Autodesk Fusion 360 part; units mm, degrees
(part 6 of 6)
sketch "Sketch8" plane through (0, -4, 0) normal (0, -1, 0) x (1, 0, 0)
  line L0 (88.7705, -19.8875) -> (88.7705, -2.0326)
  line L1 (88.7705, -2.0326) -> (97.8711, -2.0326)
  line L2 (97.8711, -2.0326) -> (97.8711, -1.7823)
  line L3 (97.8711, -1.7823) -> (111.87, -1.7823)
  line L4 (111.87, -1.7823) -> (111.87, -2.0326)
  line L5 (111.87, -2.0326) -> (120.971, -2.0326)
  line L6 (120.971, -2.0326) -> (120.971, -19.8875)
  line L7 (120.971, -19.8875) -> (88.7705, -19.8875)
  line L8 (26.1455, -15.7827) -> (26.1455, -17.7817)
  line L9 (26.1455, -17.7817) -> (12.146, -17.7817)
  line L10 (12.146, -17.7817) -> (12.146, -15.7827)
  line L11 (12.146, -15.7827) -> (11.3454, -15.7827)
  line L12 (11.3454, -15.7827) -> (11.3454, -12.6821)
  line L13 (11.3454, -12.6821) -> (12.146, -12.6821)
  line L14 (12.146, -12.6821) -> (12.146, -6.8819)
  line L15 (12.146, -6.8819) -> (11.3454, -6.8819)
  line L16 (11.3454, -6.8819) -> (11.3454, -3.7827)
  line L17 (11.3454, -3.7827) -> (12.146, -3.7827)
  line L18 (12.146, -3.7827) -> (12.146, -1.7823)
  line L19 (12.146, -1.7823) -> (26.1455, -1.7823)
  line L20 (26.1455, -1.7823) -> (26.1455, -3.7827)
  line L21 (26.1455, -3.7827) -> (26.9462, -3.7827)
  line L22 (26.9462, -3.7827) -> (26.9462, -6.8819)
  line L23 (26.9462, -6.8819) -> (26.1455, -6.8819)
  line L24 (26.1455, -6.8819) -> (26.1455, -12.6821)
  line L25 (26.1455, -12.6821) -> (26.9462, -12.6821)
  line L26 (26.9462, -12.6821) -> (26.9462, -15.7827)
  line L27 (26.9462, -15.7827) -> (26.1455, -15.7827)
  line L28 (73.7704, -34.8327) -> (73.7704, -36.8316)
  line L29 (73.7704, -36.8316) -> (59.7711, -36.8316)
  line L30 (59.7711, -36.8316) -> (59.7711, -34.8327)
  line L31 (59.7711, -34.8327) -> (58.9703, -34.8327)
  line L32 (58.9703, -34.8327) -> (58.9703, -31.7321)
  line L33 (58.9703, -31.7321) -> (59.7711, -31.7321)
  line L34 (59.7711, -31.7321) -> (59.7711, -25.9319)
  line L35 (59.7711, -25.9319) -> (58.9703, -25.9319)
  line L36 (58.9703, -25.9319) -> (58.9703, -22.8327)
  line L37 (58.9703, -22.8327) -> (59.7711, -22.8327)
  line L38 (59.7711, -22.8327) -> (59.7711, -20.8323)
  line L39 (59.7711, -20.8323) -> (73.7704, -20.8323)
  line L40 (73.7704, -20.8323) -> (73.7704, -22.8327)
  line L41 (73.7704, -22.8327) -> (74.5712, -22.8327)
  line L42 (74.5712, -22.8327) -> (74.5712, -25.9319)
  line L43 (74.5712, -25.9319) -> (73.7704, -25.9319)
  line L44 (73.7704, -25.9319) -> (73.7704, -31.7321)
  line L45 (73.7704, -31.7321) -> (74.5712, -31.7321)
  line L46 (74.5712, -31.7321) -> (74.5712, -34.8327)
  line L47 (74.5712, -34.8327) -> (73.7704, -34.8327)
  line L48 (174.071, -41.8828) -> (174.071, -39.8824)
  line L49 (174.071, -39.8824) -> (188.07, -39.8824)
  line L50 (188.07, -39.8824) -> (188.07, -41.8828)
  line L51 (188.07, -41.8828) -> (188.871, -41.8828)
  line L52 (188.871, -41.8828) -> (188.871, -44.982)
  line L53 (188.871, -44.982) -> (188.07, -44.982)
  line L54 (188.07, -44.982) -> (188.07, -50.782)
  line L55 (188.07, -50.782) -> (188.871, -50.782)
  line L56 (188.871, -50.782) -> (188.871, -53.8826)
  line L57 (188.871, -53.8826) -> (188.07, -53.8826)
  line L58 (188.07, -53.8826) -> (188.07, -55.8816)
  line L59 (188.07, -55.8816) -> (174.071, -55.8816)
  line L60 (174.071, -55.8816) -> (174.071, -53.8826)
  line L61 (174.071, -53.8826) -> (173.27, -53.8826)
  line L62 (173.27, -53.8826) -> (173.27, -50.782)
  line L63 (173.27, -50.782) -> (174.071, -50.782)
  line L64 (174.071, -50.782) -> (174.071, -44.982)
  line L65 (174.071, -44.982) -> (173.27, -44.982)
  line L66 (173.27, -44.982) -> (173.27, -41.8828)
  line L67 (173.27, -41.8828) -> (174.071, -41.8828)
  line L68 (16.6205, -53.8826) -> (16.6205, -55.8816)
  line L69 (16.6205, -55.8816) -> (2.621, -55.8816)
  line L70 (2.621, -55.8816) -> (2.621, -53.8826)
  line L71 (2.621, -53.8826) -> (1.8204, -53.8826)
  line L72 (1.8204, -53.8826) -> (1.8204, -50.782)
  line L73 (1.8204, -50.782) -> (2.621, -50.782)
  line L74 (2.621, -50.782) -> (2.621, -44.982)
  line L75 (2.621, -44.982) -> (1.8204, -44.982)
  line L76 (1.8204, -44.982) -> (1.8204, -41.8828)
  line L77 (1.8204, -41.8828) -> (2.621, -41.8828)
  line L78 (2.621, -41.8828) -> (2.621, -39.8824)
  line L79 (2.621, -39.8824) -> (16.6205, -39.8824)
  line L80 (16.6205, -39.8824) -> (16.6205, -41.8828)
  line L81 (16.6205, -41.8828) -> (17.4212, -41.8828)
  line L82 (17.4212, -41.8828) -> (17.4212, -44.982)
  line L83 (17.4212, -44.982) -> (16.6205, -44.982)
  line L84 (16.6205, -44.982) -> (16.6205, -50.782)
  line L85 (16.6205, -50.782) -> (17.4212, -50.782)
  line L86 (17.4212, -50.782) -> (17.4212, -53.8826)
  line L87 (17.4212, -53.8826) -> (16.6205, -53.8826)
  line L88 (59.7711, -41.8828) -> (59.7711, -39.8824)
  line L89 (59.7711, -39.8824) -> (73.7704, -39.8824)
  line L90 (73.7704, -39.8824) -> (73.7704, -41.8828)
  line L91 (73.7704, -41.8828) -> (74.5712, -41.8828)
  line L92 (74.5712, -41.8828) -> (74.5712, -44.982)
  line L93 (74.5712, -44.982) -> (73.7704, -44.982)
  line L94 (73.7704, -44.982) -> (73.7704, -50.782)
  line L95 (73.7704, -50.782) -> (74.5712, -50.782)
  line L96 (74.5712, -50.782) -> (74.5712, -53.8826)
  line L97 (74.5712, -53.8826) -> (73.7704, -53.8826)
  line L98 (73.7704, -53.8826) -> (73.7704, -55.8816)
  line L99 (73.7704, -55.8816) -> (59.7711, -55.8816)
  line L100 (59.7711, -55.8816) -> (59.7711, -53.8826)
  line L101 (59.7711, -53.8826) -> (58.9703, -53.8826)
  line L102 (58.9703, -53.8826) -> (58.9703, -50.782)
  line L103 (58.9703, -50.782) -> (59.7711, -50.782)
  line L104 (59.7711, -50.782) -> (59.7711, -44.982)
  line L105 (59.7711, -44.982) -> (58.9703, -44.982)
  line L106 (58.9703, -44.982) -> (58.9703, -41.8828)
  line L107 (58.9703, -41.8828) -> (59.7711, -41.8828)
  line L108 (135.971, -41.8828) -> (135.971, -39.8824)
  line L109 (135.971, -39.8824) -> (149.97, -39.8824)
  line L110 (149.97, -39.8824) -> (149.97, -41.8828)
  line L111 (149.97, -41.8828) -> (150.771, -41.8828)
  line L112 (150.771, -41.8828) -> (150.771, -44.982)
  line L113 (150.771, -44.982) -> (149.97, -44.982)
  line L114 (149.97, -44.982) -> (149.97, -50.782)
  line L115 (149.97, -50.782) -> (150.771, -50.782)
  line L116 (150.771, -50.782) -> (150.771, -53.8826)
  line L117 (150.771, -53.8826) -> (149.97, -53.8826)
  line L118 (149.97, -53.8826) -> (149.97, -55.8816)
  line L119 (149.97, -55.8816) -> (135.971, -55.8816)
  line L120 (135.971, -55.8816) -> (135.971, -53.8826)
  line L121 (135.971, -53.8826) -> (135.17, -53.8826)
  line L122 (135.17, -53.8826) -> (135.17, -50.782)
  line L123 (135.17, -50.782) -> (135.971, -50.782)
  line L124 (135.971, -50.782) -> (135.971, -44.982)
  line L125 (135.971, -44.982) -> (135.17, -44.982)
  line L126 (135.17, -44.982) -> (135.17, -41.8828)
  line L127 (135.17, -41.8828) -> (135.971, -41.8828)
  line L128 (92.8204, -53.8826) -> (92.8204, -55.8816)
  line L129 (92.8204, -55.8816) -> (78.8211, -55.8816)
  line L130 (78.8211, -55.8816) -> (78.8211, -53.8826)
  line L131 (78.8211, -53.8826) -> (78.0203, -53.8826)
  line L132 (78.0203, -53.8826) -> (78.0203, -50.782)
  line L133 (78.0203, -50.782) -> (78.8211, -50.782)
  line L134 (78.8211, -50.782) -> (78.8211, -44.982)
  line L135 (78.8211, -44.982) -> (78.0203, -44.982)
  line L136 (78.0203, -44.982) -> (78.0203, -41.8828)
  line L137 (78.0203, -41.8828) -> (78.8211, -41.8828)
  line L138 (78.8211, -41.8828) -> (78.8211, -39.8824)
  line L139 (78.8211, -39.8824) -> (92.8204, -39.8824)
  line L140 (92.8204, -39.8824) -> (92.8204, -41.8828)
  line L141 (92.8204, -41.8828) -> (93.6198, -41.8828)
  line L142 (93.6198, -41.8828) -> (93.6198, -44.982)
  line L143 (93.6198, -44.982) -> (92.8204, -44.982)
  line L144 (92.8204, -44.982) -> (92.8204, -50.782)
  line L145 (92.8204, -50.782) -> (93.6198, -50.782)
  line L146 (93.6198, -50.782) -> (93.6198, -53.8826)
  line L147 (93.6198, -53.8826) -> (92.8204, -53.8826)
  line L148 (126.446, -3.7827) -> (126.446, -1.7823)
  line L149 (126.446, -1.7823) -> (140.445, -1.7823)
  line L150 (140.445, -1.7823) -> (140.445, -3.7827)
  line L151 (140.445, -3.7827) -> (141.246, -3.7827)
  line L152 (141.246, -3.7827) -> (141.246, -6.8819)
  line L153 (141.246, -6.8819) -> (140.445, -6.8819)
  line L154 (140.445, -6.8819) -> (140.445, -12.6821)
  line L155 (140.445, -12.6821) -> (141.246, -12.6821)
  line L156 (141.246, -12.6821) -> (141.246, -15.7827)
  line L157 (141.246, -15.7827) -> (140.445, -15.7827)
  line L158 (140.445, -15.7827) -> (140.445, -17.7817)
  line L159 (140.445, -17.7817) -> (126.446, -17.7817)
  line L160 (126.446, -17.7817) -> (126.446, -15.7827)
  line L161 (126.446, -15.7827) -> (125.645, -15.7827)
  line L162 (125.645, -15.7827) -> (125.645, -12.6821)
  line L163 (125.645, -12.6821) -> (126.446, -12.6821)
  line L164 (126.446, -12.6821) -> (126.446, -6.8819)
  line L165 (126.446, -6.8819) -> (125.645, -6.8819)
  line L166 (125.645, -6.8819) -> (125.645, -3.7827)
  line L167 (125.645, -3.7827) -> (126.446, -3.7827)
  line L168 (64.2454, -1.7823) -> (64.2454, -3.7827)
  line L169 (64.2454, -3.7827) -> (65.0462, -3.7827)
  line L170 (65.0462, -3.7827) -> (65.0462, -6.8819)
  line L171 (65.0462, -6.8819) -> (64.2454, -6.8819)
  line L172 (64.2454, -6.8819) -> (64.2454, -12.6821)
  line L173 (64.2454, -12.6821) -> (65.0462, -12.6821)
  line L174 (65.0462, -12.6821) -> (65.0462, -15.7827)
  line L175 (65.0462, -15.7827) -> (64.2454, -15.7827)
  line L176 (64.2454, -15.7827) -> (64.2454, -17.7817)
  line L177 (64.2454, -17.7817) -> (50.2461, -17.7817)
  line L178 (50.2461, -17.7817) -> (50.2461, -15.7827)
  line L179 (50.2461, -15.7827) -> (49.4453, -15.7827)
  line L180 (49.4453, -15.7827) -> (49.4453, -12.6821)
  line L181 (49.4453, -12.6821) -> (50.2461, -12.6821)
  line L182 (50.2461, -12.6821) -> (50.2461, -6.8819)
  line L183 (50.2461, -6.8819) -> (49.4453, -6.8819)
  line L184 (49.4453, -6.8819) -> (49.4453, -3.7827)
  line L185 (49.4453, -3.7827) -> (50.2461, -3.7827)
  line L186 (50.2461, -3.7827) -> (50.2461, -1.7823)
  line L187 (50.2461, -1.7823) -> (64.2454, -1.7823)
  line L188 (164.546, -17.7817) -> (164.546, -15.7827)
  line L189 (164.546, -15.7827) -> (163.745, -15.7827)
  line L190 (163.745, -15.7827) -> (163.745, -12.6821)
  line L191 (163.745, -12.6821) -> (164.546, -12.6821)
  line L192 (164.546, -12.6821) -> (164.546, -6.8819)
  line L193 (164.546, -6.8819) -> (163.745, -6.8819)
  line L194 (163.745, -6.8819) -> (163.745, -3.7827)
  line L195 (163.745, -3.7827) -> (164.546, -3.7827)
  line L196 (164.546, -3.7827) -> (164.546, -1.7823)
  line L197 (164.546, -1.7823) -> (178.545, -1.7823)
  line L198 (178.545, -1.7823) -> (178.545, -3.7827)
  line L199 (178.545, -3.7827) -> (179.346, -3.7827)
  line L200 (179.346, -3.7827) -> (179.346, -6.8819)
  line L201 (179.346, -6.8819) -> (178.545, -6.8819)
  line L202 (178.545, -6.8819) -> (178.545, -12.6821)
  line L203 (178.545, -12.6821) -> (179.346, -12.6821)
  line L204 (179.346, -12.6821) -> (179.346, -15.7827)
  line L205 (179.346, -15.7827) -> (178.545, -15.7827)
  line L206 (178.545, -15.7827) -> (178.545, -17.7817)
  line L207 (178.545, -17.7817) -> (164.546, -17.7817)
  line L208 (69.2961, -17.7817) -> (69.2961, -15.7827)
  line L209 (69.2961, -15.7827) -> (68.4953, -15.7827)
  line L210 (68.4953, -15.7827) -> (68.4953, -12.6821)
  line L211 (68.4953, -12.6821) -> (69.2961, -12.6821)
  line L212 (69.2961, -12.6821) -> (69.2961, -6.8819)
  line L213 (69.2961, -6.8819) -> (68.4953, -6.8819)
  line L214 (68.4953, -6.8819) -> (68.4953, -3.7827)
  line L215 (68.4953, -3.7827) -> (69.2961, -3.7827)
  line L216 (69.2961, -3.7827) -> (69.2961, -1.7823)
  line L217 (69.2961, -1.7823) -> (83.2954, -1.7823)
  line L218 (83.2954, -1.7823) -> (83.2954, -3.7827)
  line L219 (83.2954, -3.7827) -> (84.0962, -3.7827)
  line L220 (84.0962, -3.7827) -> (84.0962, -6.8819)
  line L221 (84.0962, -6.8819) -> (83.2954, -6.8819)
  line L222 (83.2954, -6.8819) -> (83.2954, -12.6821)
  line L223 (83.2954, -12.6821) -> (84.0962, -12.6821)
  line L224 (84.0962, -12.6821) -> (84.0962, -15.7827)
  line L225 (84.0962, -15.7827) -> (83.2954, -15.7827)
  line L226 (83.2954, -15.7827) -> (83.2954, -17.7817)
  line L227 (83.2954, -17.7817) -> (69.2961, -17.7817)
  line L228 (188.07, -20.8323) -> (188.07, -22.8327)
  line L229 (188.07, -22.8327) -> (188.871, -22.8327)
  line L230 (188.871, -22.8327) -> (188.871, -25.9319)
  line L231 (188.871, -25.9319) -> (188.07, -25.9319)
  line L232 (188.07, -25.9319) -> (188.07, -31.7321)
  line L233 (188.07, -31.7321) -> (188.871, -31.7321)
  line L234 (188.871, -31.7321) -> (188.871, -34.8327)
  line L235 (188.871, -34.8327) -> (188.07, -34.8327)
  line L236 (188.07, -34.8327) -> (188.07, -36.8316)
  line L237 (188.07, -36.8316) -> (174.071, -36.8316)
  line L238 (174.071, -36.8316) -> (174.071, -34.8327)
  line L239 (174.071, -34.8327) -> (173.27, -34.8327)
  line L240 (173.27, -34.8327) -> (173.27, -31.7321)
  line L241 (173.27, -31.7321) -> (174.071, -31.7321)
  line L242 (174.071, -31.7321) -> (174.071, -25.9319)
  line L243 (174.071, -25.9319) -> (173.27, -25.9319)
  line L244 (173.27, -25.9319) -> (173.27, -22.8327)
  line L245 (173.27, -22.8327) -> (174.071, -22.8327)
  line L246 (174.071, -22.8327) -> (174.071, -20.8323)
  line L247 (174.071, -20.8323) -> (188.07, -20.8323)
  line L248 (130.92, -39.8824) -> (130.92, -41.8828)
  line L249 (130.92, -41.8828) -> (131.721, -41.8828)
  line L250 (131.721, -41.8828) -> (131.721, -44.982)
  line L251 (131.721, -44.982) -> (130.92, -44.982)
  line L252 (130.92, -44.982) -> (130.92, -50.782)
  line L253 (130.92, -50.782) -> (131.721, -50.782)
  line L254 (131.721, -50.782) -> (131.721, -53.8826)
  line L255 (131.721, -53.8826) -> (130.92, -53.8826)
  line L256 (130.92, -53.8826) -> (130.92, -55.8816)
  line L257 (130.92, -55.8816) -> (116.92, -55.8816)
  line L258 (116.92, -55.8816) -> (116.92, -53.8826)
  line L259 (116.92, -53.8826) -> (116.119, -53.8826)
  line L260 (116.119, -53.8826) -> (116.119, -50.782)
  line L261 (116.119, -50.782) -> (116.92, -50.782)
  line L262 (116.92, -50.782) -> (116.92, -44.982)
  line L263 (116.92, -44.982) -> (116.119, -44.982)
  line L264 (116.119, -44.982) -> (116.119, -41.8828)
  line L265 (116.119, -41.8828) -> (116.92, -41.8828)
  line L266 (116.92, -41.8828) -> (116.92, -39.8824)
  line L267 (116.92, -39.8824) -> (130.92, -39.8824)
  line L268 (92.8204, -20.8323) -> (92.8204, -22.8327)
  line L269 (92.8204, -22.8327) -> (93.6198, -22.8327)
  line L270 (93.6198, -22.8327) -> (93.6198, -25.9319)
  line L271 (93.6198, -25.9319) -> (92.8204, -25.9319)
  line L272 (92.8204, -25.9319) -> (92.8204, -31.7321)
  line L273 (92.8204, -31.7321) -> (93.6198, -31.7321)
  line L274 (93.6198, -31.7321) -> (93.6198, -34.8327)
  line L275 (93.6198, -34.8327) -> (92.8204, -34.8327)
  line L276 (92.8204, -34.8327) -> (92.8204, -36.8316)
  line L277 (92.8204, -36.8316) -> (78.8211, -36.8316)
  line L278 (78.8211, -36.8316) -> (78.8211, -34.8327)
  line L279 (78.8211, -34.8327) -> (78.0203, -34.8327)
  line L280 (78.0203, -34.8327) -> (78.0203, -31.7321)
  line L281 (78.0203, -31.7321) -> (78.8211, -31.7321)
  line L282 (78.8211, -31.7321) -> (78.8211, -25.9319)
  line L283 (78.8211, -25.9319) -> (78.0203, -25.9319)
  line L284 (78.0203, -25.9319) -> (78.0203, -22.8327)
  line L285 (78.0203, -22.8327) -> (78.8211, -22.8327)
  line L286 (78.8211, -22.8327) -> (78.8211, -20.8323)
  line L287 (78.8211, -20.8323) -> (92.8204, -20.8323)
  line L288 (54.7204, -39.8824) -> (54.7204, -41.8828)
  line L289 (54.7204, -41.8828) -> (55.5212, -41.8828)
  line L290 (55.5212, -41.8828) -> (55.5212, -44.982)
  line L291 (55.5212, -44.982) -> (54.7204, -44.982)
  line L292 (54.7204, -44.982) -> (54.7204, -50.782)
  line L293 (54.7204, -50.782) -> (55.5212, -50.782)
  line L294 (55.5212, -50.782) -> (55.5212, -53.8826)
  line L295 (55.5212, -53.8826) -> (54.7204, -53.8826)
  line L296 (54.7204, -53.8826) -> (54.7204, -55.8816)
  line L297 (54.7204, -55.8816) -> (40.7211, -55.8816)
  line L298 (40.7211, -55.8816) -> (40.7211, -53.8826)
  line L299 (40.7211, -53.8826) -> (39.9203, -53.8826)
  line L300 (39.9203, -53.8826) -> (39.9203, -50.782)
  line L301 (39.9203, -50.782) -> (40.7211, -50.782)
  line L302 (40.7211, -50.782) -> (40.7211, -44.982)
  line L303 (40.7211, -44.982) -> (39.9203, -44.982)
  line L304 (39.9203, -44.982) -> (39.9203, -41.8828)
  line L305 (39.9203, -41.8828) -> (40.7211, -41.8828)
  line L306 (40.7211, -41.8828) -> (40.7211, -39.8824)
  line L307 (40.7211, -39.8824) -> (54.7204, -39.8824)
  line L308 (97.8697, -55.8816) -> (97.8697, -53.8826)
  line L309 (97.8697, -53.8826) -> (97.0703, -53.8826)
  line L310 (97.0703, -53.8826) -> (97.0703, -50.782)
  line L311 (97.0703, -50.782) -> (97.8697, -50.782)
  line L312 (97.8697, -50.782) -> (97.8697, -44.982)
  line L313 (97.8697, -44.982) -> (97.0703, -44.982)
  line L314 (97.0703, -44.982) -> (97.0703, -41.8828)
  line L315 (97.0703, -41.8828) -> (97.8697, -41.8828)
  line L316 (97.8697, -41.8828) -> (97.8697, -39.8824)
  line L317 (97.8697, -39.8824) -> (111.869, -39.8824)
  line L318 (111.869, -39.8824) -> (111.869, -41.8828)
  line L319 (111.869, -41.8828) -> (112.67, -41.8828)
  line L320 (112.67, -41.8828) -> (112.67, -44.982)
  line L321 (112.67, -44.982) -> (111.869, -44.982)
  line L322 (111.869, -44.982) -> (111.869, -50.782)
  line L323 (111.869, -50.782) -> (112.67, -50.782)
  line L324 (112.67, -50.782) -> (112.67, -53.8826)
  line L325 (112.67, -53.8826) -> (111.869, -53.8826)
  line L326 (111.869, -53.8826) -> (111.869, -55.8816)
  line L327 (111.869, -55.8816) -> (97.8697, -55.8816)
  line L328 (21.671, -55.8816) -> (21.671, -53.8826)
  line L329 (21.671, -53.8826) -> (20.8704, -53.8826)
  line L330 (20.8704, -53.8826) -> (20.8704, -50.782)
  line L331 (20.8704, -50.782) -> (21.671, -50.782)
  line L332 (21.671, -50.782) -> (21.671, -44.982)
  line L333 (21.671, -44.982) -> (20.8704, -44.982)
  line L334 (20.8704, -44.982) -> (20.8704, -41.8828)
  line L335 (20.8704, -41.8828) -> (21.671, -41.8828)
  line L336 (21.671, -41.8828) -> (21.671, -39.8824)
  line L337 (21.671, -39.8824) -> (35.6704, -39.8824)
  line L338 (35.6704, -39.8824) -> (35.6704, -41.8828)
  line L339 (35.6704, -41.8828) -> (36.4712, -41.8828)
  line L340 (36.4712, -41.8828) -> (36.4712, -44.982)
  line L341 (36.4712, -44.982) -> (35.6704, -44.982)
  line L342 (35.6704, -44.982) -> (35.6704, -50.782)
  line L343 (35.6704, -50.782) -> (36.4712, -50.782)
  line L344 (36.4712, -50.782) -> (36.4712, -53.8826)
  line L345 (36.4712, -53.8826) -> (35.6704, -53.8826)
  line L346 (35.6704, -53.8826) -> (35.6704, -55.8816)
  line L347 (35.6704, -55.8816) -> (21.671, -55.8816)
  line L348 (16.6205, -20.8323) -> (16.6205, -22.8327)
  line L349 (16.6205, -22.8327) -> (17.4212, -22.8327)
  line L350 (17.4212, -22.8327) -> (17.4212, -25.9319)
  line L351 (17.4212, -25.9319) -> (16.6205, -25.9319)
  line L352 (16.6205, -25.9319) -> (16.6205, -31.7321)
  line L353 (16.6205, -31.7321) -> (17.4212, -31.7321)
  line L354 (17.4212, -31.7321) -> (17.4212, -34.8327)
  line L355 (17.4212, -34.8327) -> (16.6205, -34.8327)
  line L356 (16.6205, -34.8327) -> (16.6205, -36.8316)
  line L357 (16.6205, -36.8316) -> (2.621, -36.8316)
  line L358 (2.621, -36.8316) -> (2.621, -34.8327)
  line L359 (2.621, -34.8327) -> (1.8204, -34.8327)
  line L360 (1.8204, -34.8327) -> (1.8204, -31.7321)
  line L361 (1.8204, -31.7321) -> (2.621, -31.7321)
  line L362 (2.621, -31.7321) -> (2.621, -25.9319)
  line L363 (2.621, -25.9319) -> (1.8204, -25.9319)
  line L364 (1.8204, -25.9319) -> (1.8204, -22.8327)
  line L365 (1.8204, -22.8327) -> (2.621, -22.8327)
  line L366 (2.621, -22.8327) -> (2.621, -20.8323)
  line L367 (2.621, -20.8323) -> (16.6205, -20.8323)
  line L368 (155.021, -55.8816) -> (155.021, -53.8826)
  line L369 (155.021, -53.8826) -> (154.22, -53.8826)
  line L370 (154.22, -53.8826) -> (154.22, -50.782)
  line L371 (154.22, -50.782) -> (155.021, -50.782)
  line L372 (155.021, -50.782) -> (155.021, -44.982)
  line L373 (155.021, -44.982) -> (154.22, -44.982)
  line L374 (154.22, -44.982) -> (154.22, -41.8828)
  line L375 (154.22, -41.8828) -> (155.021, -41.8828)
  line L376 (155.021, -41.8828) -> (155.021, -39.8824)
  line L377 (155.021, -39.8824) -> (169.02, -39.8824)
  line L378 (169.02, -39.8824) -> (169.02, -41.8828)
  line L379 (169.02, -41.8828) -> (169.821, -41.8828)
  line L380 (169.821, -41.8828) -> (169.821, -44.982)
  line L381 (169.821, -44.982) -> (169.02, -44.982)
  line L382 (169.02, -44.982) -> (169.02, -50.782)
  line L383 (169.02, -50.782) -> (169.821, -50.782)
  line L384 (169.821, -50.782) -> (169.821, -53.8826)
  line L385 (169.821, -53.8826) -> (169.02, -53.8826)
  line L386 (169.02, -53.8826) -> (169.02, -55.8816)
  line L387 (169.02, -55.8816) -> (155.021, -55.8816)
  line L388 (35.6704, -20.8323) -> (35.6704, -22.8327)
  line L389 (35.6704, -22.8327) -> (36.4712, -22.8327)
  line L390 (36.4712, -22.8327) -> (36.4712, -25.9319)
  line L391 (36.4712, -25.9319) -> (35.6704, -25.9319)
  line L392 (35.6704, -25.9319) -> (35.6704, -31.7321)
  line L393 (35.6704, -31.7321) -> (36.4712, -31.7321)
  line L394 (36.4712, -31.7321) -> (36.4712, -34.8327)
  line L395 (36.4712, -34.8327) -> (35.6704, -34.8327)
  line L396 (35.6704, -34.8327) -> (35.6704, -36.8316)
  line L397 (35.6704, -36.8316) -> (21.671, -36.8316)
  line L398 (21.671, -36.8316) -> (21.671, -34.8327)
  line L399 (21.671, -34.8327) -> (20.8704, -34.8327)
  line L400 (20.8704, -34.8327) -> (20.8704, -31.7321)
  line L401 (20.8704, -31.7321) -> (21.671, -31.7321)
  line L402 (21.671, -31.7321) -> (21.671, -25.9319)
  line L403 (21.671, -25.9319) -> (20.8704, -25.9319)
  line L404 (20.8704, -25.9319) -> (20.8704, -22.8327)
  line L405 (20.8704, -22.8327) -> (21.671, -22.8327)
  line L406 (21.671, -22.8327) -> (21.671, -20.8323)
  line L407 (21.671, -20.8323) -> (35.6704, -20.8323)
  line L408 (40.7211, -36.8316) -> (40.7211, -34.8327)
  line L409 (40.7211, -34.8327) -> (39.9203, -34.8327)
  line L410 (39.9203, -34.8327) -> (39.9203, -31.7321)
  line L411 (39.9203, -31.7321) -> (40.7211, -31.7321)
  line L412 (40.7211, -31.7321) -> (40.7211, -25.9319)
  line L413 (40.7211, -25.9319) -> (39.9203, -25.9319)
  line L414 (39.9203, -25.9319) -> (39.9203, -22.8327)
  line L415 (39.9203, -22.8327) -> (40.7211, -22.8327)
  line L416 (40.7211, -22.8327) -> (40.7211, -20.8323)
  line L417 (40.7211, -20.8323) -> (54.7204, -20.8323)
  line L418 (54.7204, -20.8323) -> (54.7204, -22.8327)
  line L419 (54.7204, -22.8327) -> (55.5212, -22.8327)
  line L420 (55.5212, -22.8327) -> (55.5212, -25.9319)
  line L421 (55.5212, -25.9319) -> (54.7204, -25.9319)
  line L422 (54.7204, -25.9319) -> (54.7204, -31.7321)
  line L423 (54.7204, -31.7321) -> (55.5212, -31.7321)
  line L424 (55.5212, -31.7321) -> (55.5212, -34.8327)
  line L425 (55.5212, -34.8327) -> (54.7204, -34.8327)
  line L426 (54.7204, -34.8327) -> (54.7204, -36.8316)
  line L427 (54.7204, -36.8316) -> (40.7211, -36.8316)
  line L428 (111.869, -20.8323) -> (111.869, -22.8327)
  line L429 (111.869, -22.8327) -> (112.67, -22.8327)
  line L430 (112.67, -22.8327) -> (112.67, -25.9319)
  line L431 (112.67, -25.9319) -> (111.869, -25.9319)
  line L432 (111.869, -25.9319) -> (111.869, -31.7321)
  line L433 (111.869, -31.7321) -> (112.67, -31.7321)
  line L434 (112.67, -31.7321) -> (112.67, -34.8327)
  line L435 (112.67, -34.8327) -> (111.869, -34.8327)
  line L436 (111.869, -34.8327) -> (111.869, -36.8316)
  line L437 (111.869, -36.8316) -> (97.8697, -36.8316)
  line L438 (97.8697, -36.8316) -> (97.8697, -34.8327)
  line L439 (97.8697, -34.8327) -> (97.0703, -34.8327)
  line L440 (97.0703, -34.8327) -> (97.0703, -31.7321)
  line L441 (97.0703, -31.7321) -> (97.8697, -31.7321)
  line L442 (97.8697, -31.7321) -> (97.8697, -25.9319)
  line L443 (97.8697, -25.9319) -> (97.0703, -25.9319)
  line L444 (97.0703, -25.9319) -> (97.0703, -22.8327)
  line L445 (97.0703, -22.8327) -> (97.8697, -22.8327)
  line L446 (97.8697, -22.8327) -> (97.8697, -20.8323)
  line L447 (97.8697, -20.8323) -> (111.869, -20.8323)
  line L448 (116.92, -36.8316) -> (116.92, -34.8327)
  line L449 (116.92, -34.8327) -> (116.119, -34.8327)
  line L450 (116.119, -34.8327) -> (116.119, -31.7321)
  line L451 (116.119, -31.7321) -> (116.92, -31.7321)
  line L452 (116.92, -31.7321) -> (116.92, -25.9319)
  line L453 (116.92, -25.9319) -> (116.119, -25.9319)
  line L454 (116.119, -25.9319) -> (116.119, -22.8327)
  line L455 (116.119, -22.8327) -> (116.92, -22.8327)
  line L456 (116.92, -22.8327) -> (116.92, -20.8323)
  line L457 (116.92, -20.8323) -> (130.92, -20.8323)
  line L458 (130.92, -20.8323) -> (130.92, -22.8327)
  line L459 (130.92, -22.8327) -> (131.721, -22.8327)
  line L460 (131.721, -22.8327) -> (131.721, -25.9319)
  line L461 (131.721, -25.9319) -> (130.92, -25.9319)
  line L462 (130.92, -25.9319) -> (130.92, -31.7321)
  line L463 (130.92, -31.7321) -> (131.721, -31.7321)
  line L464 (131.721, -31.7321) -> (131.721, -34.8327)
  line L465 (131.721, -34.8327) -> (130.92, -34.8327)
  line L466 (130.92, -34.8327) -> (130.92, -36.8316)
  line L467 (130.92, -36.8316) -> (116.92, -36.8316)
  line L468 (135.971, -36.8316) -> (135.971, -34.8327)
  line L469 (135.971, -34.8327) -> (135.17, -34.8327)
  line L470 (135.17, -34.8327) -> (135.17, -31.7321)
  line L471 (135.17, -31.7321) -> (135.971, -31.7321)
  line L472 (135.971, -31.7321) -> (135.971, -25.9319)
  line L473 (135.971, -25.9319) -> (135.17, -25.9319)
  line L474 (135.17, -25.9319) -> (135.17, -22.8327)
  line L475 (135.17, -22.8327) -> (135.971, -22.8327)
  line L476 (135.971, -22.8327) -> (135.971, -20.8323)
  line L477 (135.971, -20.8323) -> (149.97, -20.8323)
  line L478 (149.97, -20.8323) -> (149.97, -22.8327)
  line L479 (149.97, -22.8327) -> (150.771, -22.8327)
  line L480 (150.771, -22.8327) -> (150.771, -25.9319)
  line L481 (150.771, -25.9319) -> (149.97, -25.9319)
  line L482 (149.97, -25.9319) -> (149.97, -31.7321)
  line L483 (149.97, -31.7321) -> (150.771, -31.7321)
  line L484 (150.771, -31.7321) -> (150.771, -34.8327)
  line L485 (150.771, -34.8327) -> (149.97, -34.8327)
  line L486 (149.97, -34.8327) -> (149.97, -36.8316)
  line L487 (149.97, -36.8316) -> (135.971, -36.8316)
  line L488 (155.021, -36.8316) -> (155.021, -34.8327)
  line L489 (155.021, -34.8327) -> (154.22, -34.8327)
  line L490 (154.22, -34.8327) -> (154.22, -31.7321)
  line L491 (154.22, -31.7321) -> (155.021, -31.7321)
  line L492 (155.021, -31.7321) -> (155.021, -25.9319)
  line L493 (155.021, -25.9319) -> (154.22, -25.9319)
  line L494 (154.22, -25.9319) -> (154.22, -22.8327)
  line L495 (154.22, -22.8327) -> (155.021, -22.8327)
  line L496 (155.021, -22.8327) -> (155.021, -20.8323)
  line L497 (155.021, -20.8323) -> (169.02, -20.8323)
  line L498 (169.02, -20.8323) -> (169.02, -22.8327)
  line L499 (169.02, -22.8327) -> (169.821, -22.8327)
  line L500 (169.821, -22.8327) -> (169.821, -25.9319)
  line L501 (169.821, -25.9319) -> (169.02, -25.9319)
  line L502 (169.02, -25.9319) -> (169.02, -31.7321)
  line L503 (169.02, -31.7321) -> (169.821, -31.7321)
  line L504 (169.821, -31.7321) -> (169.821, -34.8327)
  line L505 (169.821, -34.8327) -> (169.02, -34.8327)
  line L506 (169.02, -34.8327) -> (169.02, -36.8316)
  line L507 (169.02, -36.8316) -> (155.021, -36.8316)
  line L508 (31.196, -3.7827) -> (31.196, -1.7823)
  line L509 (31.196, -1.7823) -> (45.1954, -1.7823)
  line L510 (45.1954, -1.7823) -> (45.1954, -3.7827)
  line L511 (45.1954, -3.7827) -> (45.9962, -3.7827)
  line L512 (45.9962, -3.7827) -> (45.9962, -6.8819)
  line L513 (45.9962, -6.8819) -> (45.1954, -6.8819)
  line L514 (45.1954, -6.8819) -> (45.1954, -12.6821)
  line L515 (45.1954, -12.6821) -> (45.9962, -12.6821)
  line L516 (45.9962, -12.6821) -> (45.9962, -15.7827)
  line L517 (45.9962, -15.7827) -> (45.1954, -15.7827)
  line L518 (45.1954, -15.7827) -> (45.1954, -17.7817)
  line L519 (45.1954, -17.7817) -> (31.196, -17.7817)
  line L520 (31.196, -17.7817) -> (31.196, -15.7827)
  line L521 (31.196, -15.7827) -> (30.3954, -15.7827)
  line L522 (30.3954, -15.7827) -> (30.3954, -12.6821)
  line L523 (30.3954, -12.6821) -> (31.196, -12.6821)
  line L524 (31.196, -12.6821) -> (31.196, -6.8819)
  line L525 (31.196, -6.8819) -> (30.3954, -6.8819)
  line L526 (30.3954, -6.8819) -> (30.3954, -3.7827)
  line L527 (30.3954, -3.7827) -> (31.196, -3.7827)
  line L528 (159.495, -1.7823) -> (159.495, -3.7827)
  line L529 (159.495, -3.7827) -> (160.296, -3.7827)
  line L530 (160.296, -3.7827) -> (160.296, -6.8819)
  line L531 (160.296, -6.8819) -> (159.495, -6.8819)
  line L532 (159.495, -6.8819) -> (159.495, -12.6821)
  line L533 (159.495, -12.6821) -> (160.296, -12.6821)
  line L534 (160.296, -12.6821) -> (160.296, -15.7827)
  line L535 (160.296, -15.7827) -> (159.495, -15.7827)
  line L536 (159.495, -15.7827) -> (159.495, -17.7817)
  line L537 (159.495, -17.7817) -> (145.496, -17.7817)
  line L538 (145.496, -17.7817) -> (145.496, -15.7827)
  line L539 (145.496, -15.7827) -> (144.695, -15.7827)
  line L540 (144.695, -15.7827) -> (144.695, -12.6821)
  line L541 (144.695, -12.6821) -> (145.496, -12.6821)
  line L542 (145.496, -12.6821) -> (145.496, -6.8819)
  line L543 (145.496, -6.8819) -> (144.695, -6.8819)
  line L544 (144.695, -6.8819) -> (144.695, -3.7827)
  line L545 (144.695, -3.7827) -> (145.496, -3.7827)
  line L546 (145.496, -3.7827) -> (145.496, -1.7823)
  line L547 (145.496, -1.7823) -> (159.495, -1.7823)
  arc A0 (190.596, -18.7817) -> (188.596, -16.7817) centre (188.596, -18.7817) ccw
  line L548 (188.596, -16.7817) -> (184.846, -16.7817)
  arc A1 (182.846, -14.7817) -> (184.846, -16.7817) centre (184.846, -14.7817) ccw
  line L549 (182.846, -14.7817) -> (182.846, -2.2564)
  arc A2 (182.846, -2.2564) -> (180.846, -0.2564) centre (180.846, -2.2564) ccw
  line L550 (180.846, -0.2564) -> (167.0351, -0.2565)
  line L551 (167.0351, -0.2565) -> (137.8078, -0.2567)
  arc A3 (9.8454, -0.2576) -> (7.8454, -2.2576) centre (9.8454, -2.2576) ccw
  line L552 (7.8454, -2.2576) -> (7.8454, -14.7817)
  arc A4 (5.8454, -16.7817) -> (7.8454, -14.7817) centre (5.8454, -14.7817) ccw
  line L553 (5.8454, -16.7817) -> (2.0951, -16.7817)
  arc A5 (2.0951, -16.7817) -> (0.0951, -18.7817) centre (2.0951, -18.7817) ccw
  line L554 (0.0951, -18.7817) -> (0.0951, -55.4069)
  line L555 (0.0951, -55.4069) -> (0.102, -55.5639)
  line L556 (0.102, -55.5639) -> (0.1199, -55.7209)
  line L557 (0.1199, -55.7209) -> (0.1502, -55.874)
  line L558 (0.1502, -55.874) -> (0.1929, -56.0268)
  line L559 (0.1929, -56.0268) -> (0.248, -56.1728)
  line L560 (0.248, -56.1728) -> (0.3128, -56.315)
  line L561 (0.3128, -56.315) -> (0.39, -56.4526)
  line L562 (0.39, -56.4526) -> (0.4768, -56.5838)
  line L563 (0.4768, -56.5838) -> (0.5746, -56.7062)
  line L564 (0.5746, -56.7062) -> (0.6808, -56.8219)
  line L565 (0.6808, -56.8219) -> (0.7965, -56.9281)
  line L566 (0.7965, -56.9281) -> (0.9192, -57.0258)
  line L567 (0.9192, -57.0258) -> (1.0501, -57.113)
  line L568 (1.0501, -57.113) -> (1.1879, -57.1899)
  line L569 (1.1879, -57.1899) -> (1.3298, -57.2548)
  line L570 (1.3298, -57.2548) -> (1.4759, -57.3098)
  line L571 (1.4759, -57.3098) -> (1.6288, -57.3525)
  line L572 (1.6288, -57.3525) -> (1.7818, -57.3828)
  line L573 (1.7818, -57.3828) -> (1.9389, -57.4008)
  line L574 (1.9389, -57.4008) -> (2.096, -57.4075)
  line L575 (2.096, -57.4075) -> (6.5216, -57.4075)
  line L576 (6.5216, -57.4075) -> (35.7006, -57.4075)
  line L577 (35.7006, -57.4075) -> (154.9924, -57.4075)
  line L578 (154.9924, -57.4075) -> (184.1714, -57.4075)
  line L579 (184.1714, -57.4075) -> (188.597, -57.4075)
  line L580 (188.597, -57.4075) -> (188.753, -57.4008)
  line L581 (188.753, -57.4008) -> (188.908, -57.3828)
  line L582 (188.908, -57.3828) -> (189.063, -57.3525)
  line L583 (189.063, -57.3525) -> (189.214, -57.3098)
  line L584 (189.214, -57.3098) -> (189.362, -57.2548)
  line L585 (189.362, -57.2548) -> (189.504, -57.1899)
  line L586 (189.504, -57.1899) -> (189.64, -57.113)
  line L587 (189.64, -57.113) -> (189.771, -57.0258)
  line L588 (189.771, -57.0258) -> (189.895, -56.9281)
  line L589 (189.895, -56.9281) -> (190.011, -56.8219)
  line L590 (190.011, -56.8219) -> (190.117, -56.7062)
  line L591 (190.117, -56.7062) -> (190.215, -56.5838)
  line L592 (190.215, -56.5838) -> (190.302, -56.4526)
  line L593 (190.302, -56.4526) -> (190.379, -56.315)
  line L594 (190.379, -56.315) -> (190.444, -56.1728)
  line L595 (190.444, -56.1728) -> (190.499, -56.0268)
  line L596 (190.499, -56.0268) -> (190.54, -55.874)
  line L597 (190.54, -55.874) -> (190.572, -55.7209)
  line L598 (190.572, -55.7209) -> (190.59, -55.5639)
  line L599 (190.59, -55.5639) -> (190.596, -55.4069)
  line L600 (190.596, -55.4069) -> (190.596, -18.7817)
  line L601 (88.7705, -2.0326) -> (96.7705, -2.0326)
  line L602 (96.7705, -2.0326) -> (96.7705, -0.257)
  line L603 (96.7705, -0.257) -> (88.7705, -0.257)
  line L604 (88.7705, -0.257) -> (88.7705, -2.0326)
  line L605 (120.971, -2.0326) -> (112.971, -2.0326)
  line L606 (112.971, -2.0326) -> (112.971, 1.3)
  line L607 (112.971, 1.3) -> (120.971, 1.3)
  line L608 (120.971, 1.3) -> (120.971, -2.0326)
  line L609 (137.8078, -0.2567) -> (52.887, -0.2573)
  line L610 (52.887, -0.2573) -> (23.4739, -0.2575)
  line L611 (23.4739, -0.2575) -> (9.8454, -0.2576)
  dimension "d56" = 8
  dimension "d60" = 8
  constraint horizontal L601
  constraint vertical L602
  constraint horizontal L603
  constraint vertical L604
  constraint coincident L0.end L1.start
  constraint horizontal L605
  constraint vertical L606
  constraint horizontal L607
  constraint vertical L608
  constraint coincident L5.end L6.start
  measures "d56" distance of L0.end L601.end
  measures "d60" distance of L5.end L605.end
extrude "Extrude9" cut sketch "Sketch8" against normal blind 3 contours L1 L601 L602 L603 L604 L609 | L5 L605 L606 L608 L609 | L606 L607 L608 L609
sketch "Sketch9" plane through (0, 0, -0.2577) normal (-0.000007, 0, 1) x (1, 0, 0.000007)
  line L0 (96.7705, -1) -> (96.7705, -4)
  line L1 (96.7705, -4) -> (112.971, -4)
  line L2 (112.971, -4) -> (112.971, -1)
  line L3 (112.971, -1) -> (120.971, -1)
  line L4 (120.971, -1) -> (120.971, -4)
  line L5 (137.8078, 0) -> (52.887, 0)
  line L6 (52.887, -4) -> (88.7705, -4)
  line L7 (88.7705, -4) -> (88.7705, -1)
  line L8 (88.7705, -1) -> (96.7705, -1)
  line L9 (84.7705, 0) -> (124.971, 0)
  line L10 (124.971, 0) -> (124.971, -4)
  line L11 (124.971, -4) -> (84.7705, -4)
  line L12 (84.7705, -4) -> (84.7705, 0)
  line L13 (120.971, -4) -> (137.8078, -4)
  line L14 (137.8078, -4) -> (137.8078, 0)
  line L15 (52.887, 0) -> (52.887, -4)
  dimension "d63" = 4
  dimension "d64" = 4
  constraint horizontal L9
  constraint vertical L10
  constraint horizontal L11
  constraint vertical L12
  constraint coincident L5 L9.start
  measures "d63" distance of L4 L10
  measures "d64" distance of L7 L12
extrude "Extrude10" add sketch "Sketch9" along normal blind 1.5 contours L0 L1 L2 L3 L4 L5 L6 L7 L8 L9 L10 L11 L12 L13 | L0 L7 L8 L11 | L2 L3 L4 L11
chamfer "Chamfer3" distance 1.5 angle 45 2 edges at (124.971, -2, 1.2432) (84.7705, -2, 1.2429)
sketch "Sketch10" plane through (0, -6, 0) normal (0, -1, 0) x (1, 0, 0)
  line L0 (29.5137, 1.7425) -> (46.8457, 1.7426)
  spline S0 degree 2 poles (46.8457, 1.7426) (44.9771, 3.6334) (44.977, 7.3123) knots 0.513915 0.513915 0.513915 1 1 1
  arc A0 (44.977, 7.3123) -> (31.3817, 7.3119) centre (38.1793, 6.8699) ccw
  spline S1 degree 2 poles (31.3817, 7.3119) (31.3818, 3.6334) (29.5137, 1.7425) knots -1 -1 -1 -0.513962 -0.513962 -0.513962
  circle A1 centre (38.1793, 7.2435) radius 2.6
  line L1 (29.7492, -59.4075) -> (12.473, -59.4075)
  spline S2 degree 2 poles (12.473, -59.4075) (14.3129, -61.2982) (14.3129, -64.9763) knots 0.514047 0.514047 0.514047 1 1 1
  arc A2 (14.3129, -64.9763) -> (27.9093, -64.9763) centre (21.1111, -64.5335) ccw
  spline S3 degree 2 poles (27.9093, -64.9763) (27.9093, -61.2982) (29.7492, -59.4075) knots -1 -1 -1 -0.514047 -0.514047 -0.514047
  circle A3 centre (21.1111, -64.9075) radius 2.6
  line L2 (143.8481, 1.7434) -> (161.1783, 1.7435)
  spline S4 degree 2 poles (161.1783, 1.7435) (159.3112, 3.6343) (159.3113, 7.3119) knots 0.514087 0.514087 0.514087 1 1 1
  arc A4 (159.3113, 7.3119) -> (145.716, 7.3123) centre (152.5137, 6.8699) ccw
  spline S5 degree 2 poles (145.716, 7.3123) (145.7159, 3.6341) (143.8481, 1.7434) knots -1 -1 -1 -0.514007 -0.514007 -0.514007
  line L3 (178.22, -59.4075) -> (160.9438, -59.4075)
  spline S6 degree 2 poles (160.9438, -59.4075) (162.7837, -61.2982) (162.7837, -64.9763) knots 0.514047 0.514047 0.514047 1 1 1
  arc A5 (162.7837, -64.9763) -> (176.3801, -64.9763) centre (169.5819, -64.5335) ccw
  spline S7 degree 2 poles (176.3801, -64.9763) (176.3801, -61.2982) (178.22, -59.4075) knots -1 -1 -1 -0.514047 -0.514047 -0.514047
  circle A6 centre (169.5819, -64.9075) radius 2.6
  circle A7 centre (152.5137, 7.2435) radius 2.6
